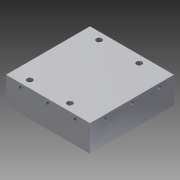
# Autodesk Inventor part: Sole_Spacer
Saved by Autodesk Inventor 2013 (Build 170138000, 138)
## iProperties
Created: 2014-02-10
Material: アセタール樹脂、白
Document SubType Name: Modeling
Designer: andou
Density: 1.425 g/cm^3
Mass: 41.9869 g
Surface Area: 89.051 cm^2
Volume: 29.4645 cm^3
Author: andou
Title: Sole_Spacer
Autodesk Inventor part; units mm, degrees
ref_plane "YZ Plane" through (0, 0, 0) normal (1, 0, 0) x (0, 1, 0)
ref_plane "XZ Plane" through (0, 0, 0) normal (0, 1, 0) x (-1, 0, 0)
ref_plane "XY Plane" through (0, 0, 0) normal (0, 0, 1) x (1, 0, 0)
sketch "スケッチ1" plane through (0, 0, 0) normal (0, 0, 1) x (1, 0, 0)
  line L0 (-23, 23) -> (23, 23)
  line L1 (23, 23) -> (23, -23)
  line L2 (23, -23) -> (-23, -23)
  line L3 (-23, -23) -> (-23, 23)
  point P0 (0, 0)
  dimension "d0" = 46
  dimension "d1" = 46
  dimension "d2" = 23
  dimension "d3" = 23
  constraints: 8 end point, 2 parallel, 1 horizontal, 1 perpendicular
  measures "d0" distance of L0.start L0.end
  measures "d1" distance of L2.end L0.start
  measures "d2" distance from line of L0 point (0, 0)
  measures "d3" distance from line of L3 point (0, 0)
extrude "押し出し1" add sketch "スケッチ1" along normal blind 14.5
sketch "スケッチ2" plane through (23, -23, 0) normal (1, 0, 0) x (0, 0, -1)
  line L0 (0, 0) -> (-14.5, 0) projected
  line L1 (0, 46) -> (-14.5, 46) projected
  circle A0 centre (-12.25, 38) radius 1
  circle A1 centre (-12.25, 8) radius 1
  circle A2 centre (-12.25, 23) radius 1
  line L2 (-14.5, 46) -> (-14.5, 0) projected
  point P0 (0, 23)
  dimension "d6" = 2
  dimension "d8" = 8
  dimension "d13" = 8
  dimension "d14" = 15
  dimension "d48" = 2.25
  dimension "d49" = 2.25
  dimension "d50" = 2.25
  constraints: 3 centre point, 2 equal radius
  measures "d6" diameter of A0
  measures "d8" distance from line of L1 A0.centre
  measures "d13" distance from line of A1.centre L0
  measures "d14" distance of A0.centre A2.centre
  measures "d48" distance from line of L2 A0.centre
  measures "d49" distance from line of L2 A2.centre
  measures "d50" distance from line of L2 A1.centre
hole "穴1" at (23, -15, 12.25) at (23, 0, 12.25) at (23, 15, 12.25) direction (-1, 0, 0) diameter 2 end through all
sketch "スケッチ3" plane through (-23, -23, 0) normal (0, -1, 0) x (1, 0, 0)
  line L0 (46, 14.5) -> (0, 14.5) projected
  line L1 (0, 0) -> (0, 14.5) projected
  line L2 (46, 0) -> (46, 14.5) projected
  circle A0 centre (8, 12.25) radius 1
  circle A1 centre (23, 12.25) radius 1
  circle A2 centre (38, 12.25) radius 1
  point P0 (23, 0)
  dimension "d22" = 2
  dimension "d23" = 2.25
  dimension "d24" = 2.25
  dimension "d25" = 2.25
  dimension "d26" = 8
  dimension "d27" = 8
  dimension "d28" = 15
  constraints: 3 centre point, 2 equal radius
  measures "d22" diameter of A0
  measures "d23" distance from line of L0 A0.centre
  measures "d24" distance from line of L0 A1.centre
  measures "d25" distance from line of A2.centre L0
  measures "d26" distance from line of L2 A2.centre
  measures "d27" distance from line of L1 A0.centre
  measures "d28" distance of A1.centre A0.centre
hole "穴2" at (-15, -23, 12.25) at (15, -23, 12.25) at (0, -23, 12.25) direction (0, 1, 0) diameter 2 end through all
thread "ねじ1" size "M2x0.4" class "6H" standard "ANSI Metric M Profile" full length
thread "ねじ2" size "M2x0.4" class "6H" standard "ANSI Metric M Profile" full length
thread "ねじ3" size "M2x0.4" class "6H" standard "ANSI Metric M Profile" full length
thread "ねじ4" size "M2x0.4" class "6H" standard "ANSI Metric M Profile" full length
thread "ねじ5" size "M2x0.4" class "6H" standard "ANSI Metric M Profile" full length
thread "ねじ6" size "M2x0.4" class "6H" standard "ANSI Metric M Profile" full length
sketch "スケッチ4" plane through (0, 0, 14.5) normal (0, 0, 1) x (1, 0, 0)
  line L0 (-23, -23) -> (-23, 23) projected
  line L1 (23, -23) -> (-23, -23) projected
  circle A0 centre (-14, 19) radius 1.5
  circle A1 centre (8, 19) radius 1.5
  circle A2 centre (-14, -19) radius 1.5
  circle A3 centre (8, -19) radius 1.5
  dimension "d51" = 3
  dimension "d52" = 22
  dimension "d53" = 22
  dimension "d54" = 38
  dimension "d55" = 38
  dimension "d88" = 9
  dimension "d89" = 9
  dimension "d90" = 4
  dimension "d91" = 4
  constraints: 4 centre point, 3 equal radius
  measures "d51" diameter of A0
  measures "d52" distance of A1.centre A0.centre
  measures "d53" distance of A2.centre A3.centre
  measures "d54" distance of A1.centre A3.centre
  measures "d55" distance of A2.centre A0.centre
  measures "d88" distance from line of L0 A2.centre
  measures "d89" distance from line of L0 A0.centre
  measures "d90" distance from line of A2.centre L1
  measures "d91" distance from line of L1 A3.centre
hole "穴3" at (-14, -19, 14.5) at (-14, 19, 14.5) at (8, -19, 14.5) at (8, 19, 14.5) direction (0, 0, -1) diameter 3 end through all
thread "ねじ7" size "M3x0.5" class "6H" standard "ANSI Metric M Profile" full length
thread "ねじ8" size "M3x0.5" class "6H" standard "ANSI Metric M Profile" full length
thread "ねじ9" size "M3x0.5" class "6H" standard "ANSI Metric M Profile" full length
thread "ねじ10" size "M3x0.5" class "6H" standard "ANSI Metric M Profile" full length
thread "ねじ11" size "M2x0.4" class "6H" standard "ANSI Metric M Profile" full length
thread "ねじ12" size "M2x0.4" class "6H" standard "ANSI Metric M Profile" full length
thread "ねじ13" size "M2x0.4" class "6H" standard "ANSI Metric M Profile" full length
thread "ねじ14" size "M2x0.4" class "6H" standard "ANSI Metric M Profile" full length
thread "ねじ15" size "M2x0.4" class "6H" standard "ANSI Metric M Profile" full length
thread "ねじ16" size "M2x0.4" class "6H" standard "ANSI Metric M Profile" full length
